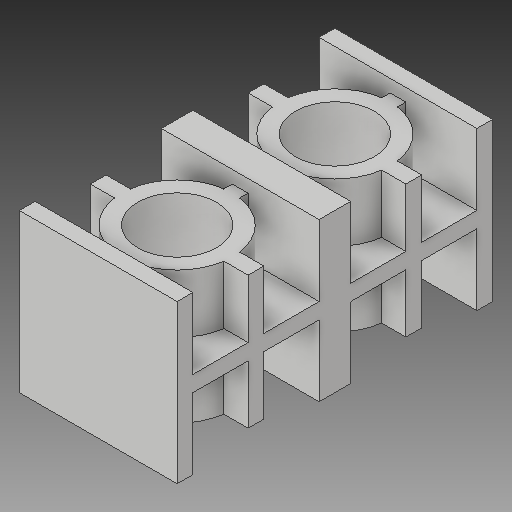
# Autodesk Inventor part: straight_beam_inner_part
Saved by Autodesk Inventor 2019 (Build 230136000, 136)
## iProperties
Created: 2019-01-31
Part Number: straight_beam_inner_part
Material: Generic
Document SubType Name: Modeling
Designer: Varga Daniel
Density: 1 g/cm^3
Appearance: Default
Author: Varga Daniel
Autodesk Inventor part; units mm, degrees
ref_plane "YZ Plane" through (0, 0, 0) normal (1, 0, 0) x (0, 1, 0)
ref_plane "XZ Plane" through (0, 0, 0) normal (0, 1, 0) x (-1, 0, 0)
derived "Base_part.ipt"
sketch "Sketch1" plane through (0, 0, 0) normal (0, 1, 0) x (-1, 0, 0)
  line L0 (5, 0) -> (25, 0)
  line L1 (30, 5) -> (30, 25)
  line L2 (25, 30) -> (5, 30)
  line L3 (0, 25) -> (0, 5)
  line L4 (5, 29) -> (25, 29)
  line L5 (29, 25) -> (29, 5)
  line L6 (25, 1) -> (5, 1)
  line L7 (1, 5) -> (1, 25)
  circle A0 centre (5, 5) radius 2.5
  circle A1 centre (5, 5) radius 3.5
  arc A2 (25, 0) -> (30, 5) centre (25, 5) ccw
  arc A3 (30, 25) -> (25, 30) centre (25, 25) ccw
  arc A4 (5, 30) -> (0, 25) centre (5, 25) ccw
  arc A5 (0, 5) -> (5, 0) centre (5, 5) ccw
  arc A6 (1, 5) -> (5, 1) centre (5, 5) ccw
  arc A7 (5, 29) -> (1, 25) centre (5, 25) ccw
  arc A8 (29, 25) -> (25, 29) centre (25, 25) ccw
  arc A9 (25, 1) -> (29, 5) centre (25, 5) ccw
  line L8 (49.1041, 15) -> (-27.081, 15) construction
  line L9 (31.1478, 10) -> (-2.4877, 10) construction
  line L10 (-2.8604, 5) -> (35.495, 5) construction
  line L11 (5, -2.5736) -> (5, 36.7522) construction
  line L12 (15, -1.4978) -> (15, 34.8784) construction
  line L13 (1.5359, 5.5) -> (1, 5.5)
  line L14 (1.5359, 4.5) -> (1.0314, 4.5)
  line L15 (28.9686, 4.5) -> (8.4641, 4.5)
  line L16 (29, 5.5) -> (8.4641, 5.5)
  line L17 (4.5, 1.5359) -> (4.5, 1.0314)
  line L18 (5.5, 1.5359) -> (5.5, 1)
  line L19 (29, 10.5) -> (1, 10.5)
  line L20 (29, 9.5) -> (1, 9.5)
  line L21 (4.5, 28.9686) -> (4.5, 10.5)
  line L22 (4.5, 9.5) -> (4.5, 8.4641)
  line L23 (5.5, 29) -> (5.5, 10.5)
  line L24 (5.5, 9.5) -> (5.5, 8.4641)
  point P0 (0, 0)
  point P1 (30, 30)
  point P2 (0, 30)
  point P3 (5, 25)
sketch "Sketch3" plane through (0, 0, 0) normal (0, 1, 0) x (-1, 0, 0)
  circle A0 centre (5, 5) radius 2.5 construction
  circle A1 centre (5, 5) radius 3.5 construction
  circle A2 centre (5, 5) radius 2.5
  circle A3 centre (5, 5) radius 3.5
  line L0 (0.3508, 5) -> (13.598, 5) construction
  line L1 (5, 15) -> (5, -1.7484) construction
  line L2 (0, 20) -> (0, 5.5)
  line L3 (10, 9) -> (10, 10)
  line L4 (10, 1) -> (0, 1)
  line L5 (0, 1) -> (0, 0)
  line L6 (0, 0) -> (10, 0)
  line L7 (10, 0) -> (10, 1)
  line L8 (10, 20) -> (10, 9)
  line L9 (0, 0) -> (0, 9)
  line L10 (8.4641, 5.5) -> (10, 5.5)
  line L11 (10, 5.5) -> (10, 4.5)
  line L12 (10, 4.5) -> (8.4641, 4.5)
  line L13 (1.5359, 5.5) -> (0, 5.5)
  line L14 (0, 5.5) -> (0, 4.5)
  line L15 (0, 4.5) -> (1.5359, 4.5)
  line L16 (5.5, 9) -> (5.5, 8.4641)
  line L17 (4.5, 1.5359) -> (4.5, 1)
  line L18 (5.5, 1.5359) -> (5.5, 1)
  line L19 (0, 9) -> (0, 10)
  line L20 (10, 20) -> (0, 20)
  line L21 (10, 10) -> (0, 10) construction
  line L22 (10, 9) -> (5.5, 9)
  line L23 (10, 11) -> (0, 11)
  line L24 (4.5, 9) -> (4.5, 8.4641)
  line L25 (10, 15) -> (0, 15) construction
  line L26 (10, 19) -> (0, 19)
  circle A4 centre (5, 15) radius 2.5
  circle A5 centre (5, 15) radius 3.5
  line L27 (5.5, 11.5359) -> (5.5, 11)
  line L28 (4.5, 11.5359) -> (4.5, 11)
  line L29 (4.5, 18.4641) -> (4.5, 19)
  line L30 (5.5, 18.4641) -> (5.5, 19)
  line L31 (1.5359, 14.5) -> (0, 14.5)
  line L32 (1.5359, 15.5) -> (0, 15.5)
  line L33 (8.4641, 15.5) -> (10, 15.5)
  line L34 (10, 14.5) -> (8.4641, 14.5)
  line L35 (10, 9) -> (10, 0)
  line L36 (5.5, 9) -> (0, 9)
  point P0 (0, 0)
  dimension "d28" = 7
  dimension "d3" = 10
  dimension "d4" = 1
  dimension "d6" = 1
  dimension "d20" = 20
  dimension "d21" = 2
  dimension "d23" = 1
  dimension "d24" = 13.2471
  dimension "d25" = 1
  dimension "d26" = 5
  dimension "d27" = 7
  dimension "d29" = 5
  dimension "d30" = 1
  constraints: 70 end point, 16 point on line, 11 parallel, 9 collinear, 5 horizontal, 5 perpendicular, 5 vertical, 4 coincident, 3 midpoint, 2 centre point, 1 concentric, 52 other
  measures "d3" distance of the line from the sketch origin of L3
  measures "d4" distance between parallel lines of L4 L6
  measures "d6" distance between parallel lines of L10 L12
  measures "d20" distance between parallel lines of L6 L20
  measures "d21" distance between parallel lines of L22 L23
  measures "d23" distance between parallel lines of L17 L18
  measures "d24" distance of L0.start L0.end
  measures "d25" distance between parallel lines of L20 L26
  measures "d26" diameter of A0
  measures "d27" diameter of A1
  measures "d29" diameter of A4
  measures "d30" distance between parallel lines of L32 L31
ref_plane "Work Plane2" through (0, 0, 20) normal (0, 1, 0) x (0, 0, -1)
extrude "Extrusion7" add sketch "Sketch3" along normal blind 5 contours L36 L2 L23 L8 L3 L22 | L4 L7 L6 L5 | L26 L2 L20 L8
extrude "Extrusion8" add sketch "Sketch3" against normal blind 5 contours L36 L2 L23 L8 L3 L22 | L4 L7 L6 L5 | L26 L2 L20 L8
extrude "Extrusion9" add sketch "Sketch3" along normal blind 4.2 contours A3 | A3 L10 L11 L12 | A3 L24 L36 L16 | L18 L4 L17 A3 | A3 L15 L9 L13 | L34 A5 L33 L8 | L23 L28 A5 L27 | A5 | L2 L32 A5 L31 | L30 A5 L29 L26
extrude "Extrusion10" add sketch "Sketch3" against normal blind 4.2 contours A3 | A3 L10 L11 L12 | A3 L24 L36 L16 | L18 L4 L17 A3 | A3 L15 L9 L13 | L34 A5 L33 L8 | L23 L28 A5 L27 | A5 | L2 L32 A5 L31 | L30 A5 L29 L26
extrude "Extrusion11" add sketch "Sketch3" along normal blind 0.5 contours A3 L16 L22 L35 L10 | L12 L35 L4 L18 A3 | A3 L13 L2 L36 L24 | L17 L4 L9 L15 A3 | L23 L27 A5 L34 L8 | L2 L31 A5 L28 L23 | L33 A5 L30 L26 L8 | L2 L26 L29 A5 L32
extrude "Extrusion12" add sketch "Sketch3" against normal blind 0.5 contours A3 L16 L22 L35 L10 | L12 L35 L4 L18 A3 | A3 L13 L2 L36 L24 | L17 L4 L9 L15 A3 | L23 L27 A5 L34 L8 | L2 L31 A5 L28 L23 | L33 A5 L30 L26 L8 | L2 L26 L29 A5 L32
equation "\"d28\" = d27"
equation "\"d4\" = Wall_thickness"
equation "\"d6\" = Inner_route_thickness"
equation "\"d21\" = 2 * Wall_thickness"
equation "\"d23\" = Inner_route_thickness"
equation "\"d25\" = Wall_thickness"
equation "\"d29\" = d26"
equation "\"d30\" = Inner_route_thickness"
equation "\"d31\" = 0.5 * Overall_height"
equation "\"d33\" = 0.5 * Overall_height"
equation "\"d35\" = 0.5 * Hole_height"
equation "\"d37\" = 0.5 * Hole_height"
equation "\"d39\" = 0.5 * Inner_thickness"
equation "\"d41\" = 0.5 * Inner_thickness"
equation "\"Wall_thickness\" = 1"
equation "\"Inner_route_thickness\" = 1"
equation "\"Overall_height\" = 10"
equation "\"Hole_height\" = 8.4"
equation "\"Inner_thickness\" = 1"
body "Solid2"
